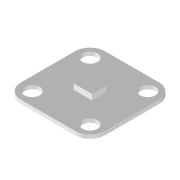
# Autodesk Inventor part: 00_AS5600_rotational_encoder_i2c
Saved by Autodesk Inventor 2022 (Build 260153000, 153)
## iProperties
Created: 2023-07-28
Part Number: 00_AS5600_rotational_encoder_i2c
Material: Generisch
Document SubType Name: Modeling
Designer: diederichbenedict
Density: 1 g/cm^3
Appearance: Vorgabe
Author: diederichbenedict
Autodesk Inventor part; units mm, degrees
ref_plane "YZ Plane" through (0, 0, 0) normal (1, 0, 0) x (0, 1, 0)
ref_plane "XZ Plane" through (0, 0, 0) normal (0, 1, 0) x (-1, 0, 0)
ref_plane "XY Plane" through (0, 0, 0) normal (0, 0, 1) x (1, 0, 0)
sketch "Skizze1" plane through (0, 0, 0) normal (0, 1, 0) x (-1, 0, 0)
  line L0 (7.25, -11.25) -> (-7.25, -11.25)
  line L1 (-11.25, -7.25) -> (-11.25, 7.25)
  line L2 (-7.25, 11.25) -> (7.25, 11.25)
  line L3 (11.25, 7.25) -> (11.25, -7.25)
  line L4 (11.25, -11.25) -> (-11.25, 11.25) construction
  line L5 (-11.25, -11.25) -> (11.25, 11.25) construction
  arc A0 (-7.25, 11.25) -> (-11.25, 7.25) centre (-7.25, 7.25) ccw
  arc A1 (11.25, 7.25) -> (7.25, 11.25) centre (7.25, 7.25) ccw
  arc A2 (7.25, -11.25) -> (11.25, -7.25) centre (7.25, -7.25) ccw
  arc A3 (-11.25, -7.25) -> (-7.25, -11.25) centre (-7.25, -7.25) ccw
  point P0 (0, 0)
  dimension "d0" = 22.5
  dimension "d1" = 22.5
  dimension "d2" = 4
  constraints: 12 end point, 8 point on circle, 8 point on line, 8 tangent, 4 centre point, 3 equal radius, 2 midpoint, 2 parallel, 1 horizontal, 1 perpendicular
  measures "d0" distance of L4.end L5.end
  measures "d1" distance of L5.start L4.end
  measures "d2" radius of A0
extrude "Extrusion1" add sketch "Skizze1" along normal blind 1
sketch "Skizze2" plane through (0, 1, 0) normal (0, 1, 0) x (1, 0, 0)
  line L0 (-7.25, -11.25) -> (7.25, -11.25) projected
  arc A0 (7.25, -11.25) -> (11.25, -7.25) centre (7.25, -7.25) ccw projected
  line L1 (11.25, -7.25) -> (11.25, 7.25) projected
  arc A1 (11.25, 7.25) -> (7.25, 11.25) centre (7.25, 7.25) ccw projected
  line L2 (7.25, 11.25) -> (-7.25, 11.25) projected
  arc A2 (-7.25, 11.25) -> (-11.25, 7.25) centre (-7.25, 7.25) ccw projected
  line L3 (-11.25, 7.25) -> (-11.25, -7.25) projected
  arc A3 (-11.25, -7.25) -> (-7.25, -11.25) centre (-7.25, -7.25) ccw projected
  line L4 (2.45, -1.9) -> (-2.45, -1.9)
  line L5 (-2.45, -1.9) -> (-2.45, 1.9)
  line L6 (-2.45, 1.9) -> (2.45, 1.9)
  line L7 (2.45, 1.9) -> (2.45, -1.9)
  line L8 (2.45, -1.9) -> (-2.45, 1.9) construction
  line L9 (-2.45, -1.9) -> (2.45, 1.9) construction
  point P0 (0, 0)
  dimension "d5" = 4.9
  dimension "d6" = 3.8
  constraints: 12 end point, 2 midpoint, 2 parallel, 1 horizontal, 1 perpendicular
  measures "d5" distance of L5.end L6.end
  measures "d6" distance of L4.end L5.end
extrude "Extrusion2" add sketch "Skizze2" along normal blind 1.5 contours L4 L5 L6 L7
sketch "Skizze3" plane through (0, 1, 0) normal (0, 1, 0) x (1, 0, 0)
  line L0 (2.45, 1.9) -> (2.45, -1.9) projected
  line L1 (2.45, -1.9) -> (-2.45, -1.9) projected
  line L2 (-2.45, -1.9) -> (-2.45, 1.9) projected
  line L3 (-2.45, 1.9) -> (2.45, 1.9) projected
  line L4 (-7.25, -11.25) -> (7.25, -11.25) projected
  arc A0 (7.25, -11.25) -> (11.25, -7.25) centre (7.25, -7.25) ccw projected
  line L5 (11.25, -7.25) -> (11.25, 7.25) projected
  arc A1 (11.25, 7.25) -> (7.25, 11.25) centre (7.25, 7.25) ccw projected
  line L6 (7.25, 11.25) -> (-7.25, 11.25) projected
  arc A2 (-7.25, 11.25) -> (-11.25, 7.25) centre (-7.25, 7.25) ccw projected
  line L7 (-11.25, 7.25) -> (-11.25, -7.25) projected
  arc A3 (-11.25, -7.25) -> (-7.25, -11.25) centre (-7.25, -7.25) ccw projected
  line L8 (-7.75, 7.75) -> (7.75, 7.75) construction
  line L9 (7.75, 7.75) -> (7.75, -7.75) construction
  line L10 (7.75, -7.75) -> (-7.75, -7.75) construction
  line L11 (-7.75, -7.75) -> (-7.75, 7.75) construction
  line L12 (-7.75, 7.75) -> (7.75, -7.75) construction
  line L13 (7.75, 7.75) -> (-7.75, -7.75) construction
  point P0 (0, 0)
  dimension "d9" = 15.5
  dimension "d10" = 15.5
  constraints: 12 end point, 4 coincident, 2 midpoint, 2 parallel, 1 horizontal, 1 perpendicular
  measures "d9" distance of L9.end L10.end
  measures "d10" distance of L8.end L9.end
hole "Bohrung1" at (7.75, 1, 7.75) at (-7.75, 1, 7.75) at (-7.75, 1, -7.75) at (7.75, 1, -7.75) direction (0, -1, 0) diameter 4 depth 3 tip angle 118
sketch "Skizze4" plane through (0, 0, 0) normal (0, -1, 0) x (1, 0, 0)
  circle A0 centre (0, 0) radius 2.2643
  constraints: 1 centre point, 1 coincident
extrude "Extrusion3" cut sketch "Skizze4" against normal blind 0.5
